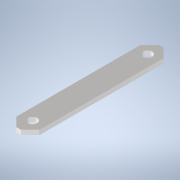
# Autodesk Inventor part: Schenkel
Saved by Autodesk Inventor 2022 (Build 260153000, 153)
## iProperties
Created: 2022-06-01
Part Number: Schenkel
Material: Generisch
Document SubType Name: Modeling
Designer: kaebi
Density: 1 g/cm^3
Appearance: Vorgabe
Author: kaebi
Autodesk Inventor part; units mm, degrees
ref_plane "YZ Plane" through (0, 0, 0) normal (1, 0, 0) x (0, 1, 0)
ref_plane "XZ Plane" through (0, 0, 0) normal (0, 1, 0) x (-1, 0, 0)
ref_plane "XY Plane" through (0, 0, 0) normal (0, 0, 1) x (1, 0, 0)
sketch "Skizze1" plane through (0, 0, 0) normal (0, 1, 0) x (-1, 0, 0)
  line L0 (-2.5, 15.5) -> (2.5, 15.5)
  line L1 (2.5, 15.5) -> (2.5, -15.5)
  line L2 (2.5, -15.5) -> (-2.5, -15.5)
  line L3 (-2.5, -15.5) -> (-2.5, 15.5)
  line L4 (-2.5, 15.5) -> (2.5, -15.5) construction
  line L5 (2.5, 15.5) -> (-2.5, -15.5) construction
  circle A0 centre (0, 12.5) radius 1
  circle A1 centre (0, -12.5) radius 1
  line L6 (3.5, 0) -> (-3.5, 0) projected
  point P0 (0, 0)
  point P1 (0, 0)
  dimension "d1" = 5
  dimension "d2" = 3
  dimension "d3" = 2
  dimension "d9" = 25
  constraints: 12 end point, 3 midpoint, 2 centre point, 2 parallel, 1 equal radius, 1 horizontal, 1 perpendicular, 1 vertical alignment, 1 other
  measures "d1" distance of L1.end L2.end
  measures "d2" distance from line of L0 A0.centre
  measures "d3" diameter of A0
  measures "d9" distance of A1.centre A0.centre
extrude "Extrusion1" add sketch "Skizze1" along normal mid plane 1
chamfer "Fase1" distance 2 angle 45 4 edges at (-2.5, 0, 15.5) (2.5, 0, 15.5) (-2.5, 0, -15.5) (2.5, 0, -15.5)
